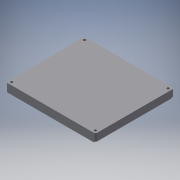
# Autodesk Inventor part: case rear
Saved by Autodesk Inventor 2018 (Build 220112000, 112)
## iProperties
Created: 2017-11-16
Part Number: case rear
Material: ABS-Kunststoff
Document SubType Name: Modeling
Designer: Till
Density: 1.06 g/cm^3
Appearance: Rot
Author: Till
Autodesk Inventor part; units mm, degrees
ref_plane "YZ Plane" through (0, 0, 0) normal (1, 0, 0) x (0, 1, 0)
ref_plane "XZ Plane" through (0, 0, 0) normal (0, 1, 0) x (-1, 0, 0)
ref_plane "XY Plane" through (0, 0, 0) normal (0, 0, 1) x (1, 0, 0)
sketch "Skizze1" plane through (0, 0, 0) normal (0, 0, 1) x (1, 0, 0)
  line L0 (52.3, 47.7) -> (-52.3, 47.7) projected
  arc A0 (-52.3, 47.7) -> (-54.3, 45.7) centre (-52.3, 45.7) ccw projected
  line L1 (54.3, 23.5) -> (54.3, 45.7) projected
  line L2 (-54.3, 45.7) -> (-54.3, -45.7) projected
  line L3 (-52.3, -47.7) -> (52.3, -47.7) projected
  arc A1 (-54.3, -45.7) -> (-52.3, -47.7) centre (-52.3, -45.7) ccw projected
  circle A2 centre (-50.8, -44.2) radius 1.5 projected
  circle A3 centre (50.8, 44.2) radius 1.5 projected
  arc A4 (52.3, -47.7) -> (54.3, -45.7) centre (52.3, -45.7) ccw projected
  line L4 (54.3, -45.7) -> (54.3, -8.7) projected
  line L5 (54.3, 23.5) -> (54.3, -8.7) projected
  arc A5 (54.3, 45.7) -> (52.3, 47.7) centre (52.3, 45.7) ccw projected
  circle A6 centre (-50.8, 44.2) radius 1.5 projected
  circle A7 centre (50.8, -44.2) radius 1.5 projected
  point P0 (0, 0)
extrude "Extrusion1" add sketch "Skizze1" along normal blind 10
sketch "Skizze2" plane through (0, 0, 0) normal (0, 0, -1) x (-1, 0, 0)
  line L0 (53.1, -44.5) -> (53.1, 44.5) projected
  line L1 (51.1, 46.5) -> (-51.1, 46.5) projected
  line L2 (-53.1, 44.5) -> (-53.1, -44.5) projected
  line L3 (-51.1, -46.5) -> (51.1, -46.5) projected
  line L4 (-51.3, -46.7) -> (51.3, -46.7)
  line L5 (53.3, -44.7) -> (53.3, 44.7)
  line L6 (51.3, 46.7) -> (-51.3, 46.7)
  line L7 (-53.3, 44.7) -> (-53.3, -44.7)
  line L8 (-53.3, -46.7) -> (53.3, 46.7) construction
  line L9 (53.3, -46.7) -> (-53.3, 46.7) construction
  arc A0 (53.3, 44.7) -> (51.3, 46.7) centre (51.3, 44.7) ccw
  arc A1 (-51.3, 46.7) -> (-53.3, 44.7) centre (-51.3, 44.7) ccw
  arc A2 (-53.3, -44.7) -> (-51.3, -46.7) centre (-51.3, -44.7) ccw
  arc A3 (51.3, -46.7) -> (53.3, -44.7) centre (51.3, -44.7) ccw
  line L10 (-56.7586, -49.6784) -> (56.7586, -49.6784)
  line L11 (56.7586, -49.6784) -> (56.7586, 49.6784)
  line L12 (56.7586, 49.6784) -> (-56.7586, 49.6784)
  line L13 (-56.7586, 49.6784) -> (-56.7586, -49.6784)
  line L14 (-56.7586, -49.6784) -> (56.7586, 49.6784) construction
  line L15 (56.7586, -49.6784) -> (-56.7586, 49.6784) construction
  point P0 (0, 0)
  dimension "d2" = 0.2
  dimension "d3" = 0.2
  dimension "d4" = 2
  constraints: 24 end point, 8 point on circle, 8 point on line, 8 tangent, 4 centre point, 4 midpoint, 4 parallel, 3 equal radius, 2 horizontal, 2 perpendicular
  measures "d2" distance between parallel lines of L1 L6
  measures "d3" distance between parallel lines of L0 L5
  measures "d4" radius of A0
extrude "Extrusion2" cut sketch "Skizze2" against normal blind 1.85
sketch "Skizze3" plane through (0, 0, 0) normal (0, 0, -1) x (-1, 0, 0)
  line L0 (-50.7142, 40.2858) -> (-46.8858, 44.1142) projected
  arc A0 (-45.4716, 44.7) -> (-46.8858, 44.1142) centre (-45.4716, 42.7) ccw projected
  line L1 (-45.4716, 44.7) -> (45.4716, 44.7) projected
  arc A1 (-50.7142, 40.2858) -> (-51.3, 38.8716) centre (-49.3, 38.8716) ccw projected
  line L2 (-51.3, -38.8716) -> (-51.3, 38.8716) projected
  line L3 (50.7142, -40.2858) -> (46.8858, -44.1142) projected
  arc A2 (50.7142, -40.2858) -> (51.3, -38.8716) centre (49.3, -38.8716) ccw projected
  line L4 (51.3, 38.8716) -> (51.3, -38.8716) projected
  arc A3 (45.4716, -44.7) -> (46.8858, -44.1142) centre (45.4716, -42.7) ccw projected
  line L5 (45.4716, -44.7) -> (-45.4716, -44.7) projected
  arc A4 (51.3, 38.8716) -> (50.7142, 40.2858) centre (49.3, 38.8716) ccw projected
  line L6 (46.8858, 44.1142) -> (50.7142, 40.2858) projected
  arc A5 (46.8858, 44.1142) -> (45.4716, 44.7) centre (45.4716, 42.7) ccw projected
  arc A6 (-46.8858, -44.1142) -> (-45.4716, -44.7) centre (-45.4716, -42.7) ccw projected
  line L7 (-46.8858, -44.1142) -> (-50.7142, -40.2858) projected
  arc A7 (-51.3, -38.8716) -> (-50.7142, -40.2858) centre (-49.3, -38.8716) ccw projected
  circle A8 centre (-50.8, -44.2) radius 1.5 projected
  circle A9 centre (-50.8, 44.2) radius 1.5 projected
  circle A10 centre (50.8, 44.2) radius 1.5 projected
  circle A11 centre (50.8, -44.2) radius 1.5 projected
  point P0 (0, 0)
extrude "Extrusion3" cut sketch "Skizze3" against normal blind 8 contours L0 A0 L1 A5 L6 A4 L4 A2 L3 A3 L5 A6 L7 A7 L2 A1
